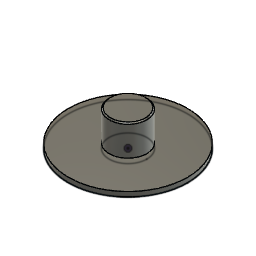
BearingBaseMount (Autodesk Fusion 360 design; units mm, degrees)
Autodesk Fusion 360 part; units mm, degrees
sketch "Sketch1" plane through (0, 0, 0) normal (0, 1, 0) x (1, 0, 0)
  circle A0 centre (0, 0) radius 12.7
  circle A1 centre (0, 0) radius 4
  dimension "d1" = 25.4
  dimension "d4" = 8
  constraint coincident A0.centre A1.centre
  constraint concentric A0 A1
  measures "d1" diameter of A0
  measures "d4" diameter of A1
extrude "Extrude1" add sketch "Sketch1" along normal blind 1
extrude "Extrude2" add sketch "Sketch1" along normal blind 7.5 contours A1
chamfer "Chamfer1" distance 0.25 angle 45 1 edges at (-3.7293, 7.5, 1.4465)
equation "d5 = 10.5 mm - 3 mm"
